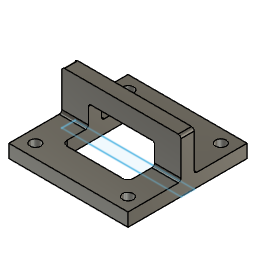
tesion holder v1 (Autodesk Fusion 360 design; units mm, degrees)
Autodesk Fusion 360 part; units mm, degrees
sketch "Sketch1" plane through (0, 0, 0) normal (0, 0, 1) x (1, 0, 0)
  line L0 (0, 0) -> (45, 0)
  line L1 (45, 0) -> (45, 45)
  line L2 (45, 45) -> (0, 45)
  line L3 (0, 45) -> (0, 0)
  line L4 (10, 35) -> (35, 35)
  line L5 (35, 35) -> (35, 10)
  line L6 (35, 10) -> (10, 10)
  line L7 (10, 10) -> (10, 35)
  dimension "d1" = 45
  dimension "d2" = 45
  constraint coincident L0.start L3.end
  constraint horizontal L0
  constraint perpendicular L0 L1
  constraint perpendicular L1 L2
  constraint perpendicular L0 L3
  constraint horizontal L4
  constraint perpendicular L4 L5
  constraint perpendicular L5 L6
  constraint perpendicular L4 L7
  measures "d1" distance of L0.start L0.end
  measures "d2" distance of L0.end L1.end
extrude "Extrude1" add sketch "Sketch1" along normal blind 5
hole "Hole1" at (5.1121, 40.0517, 5) direction (0, 0, -1) diameter 4 depth 10 tip angle 180
hole "Hole2" at (4.9695, 5.025, 5) direction (0, 0, -1) diameter 4 depth 6 tip angle 180
hole "Hole3" at (39.9447, 5.025, 5) direction (0, 0, -1) diameter 4 depth 6 tip angle 180
hole "Hole4" at (40.0084, 40.0762, 5) direction (0, 0, -1) diameter 4 depth 6 tip angle 180
sketch "Sketch2" plane through (0, 0, 0) normal (0, 0, 1) x (1, 0, 0)
  line L0 (45, 25) -> (45, 20)
  line L1 (45, 20) -> (0, 20)
  line L2 (0, 20) -> (0, 25)
  line L3 (0, 25) -> (0, 20)
  line L4 (0, 25) -> (45, 25)
  constraint vertical L0
  constraint perpendicular L0 L1
  constraint perpendicular L1 L2
  constraint perpendicular L0 L4
extrude "Extrude2" add sketch "Sketch2" along normal blind 20
sketch "Sketch4" plane through (0, 25, 0) normal (0, 1, 0) x (-1, 0, 0)
  line L0 (-45, 5) -> (-35, 5)
  line L1 (-35, 5) -> (-35, 0)
  line L2 (-35, 0) -> (-10, 0)
  line L3 (-10, 0) -> (-10, 5)
  line L4 (-10, 5) -> (0, 5)
  line L5 (0, 5) -> (0, 20)
  line L6 (0, 20) -> (-45, 20)
  line L7 (-45, 20) -> (-45, 5)
  line L8 (-10, 0) -> (-35, 0)
  line L9 (-35, 0) -> (-35, 13.0137)
  line L10 (-35, 13.0137) -> (-10, 13.0137)
  line L11 (-10, 13.0137) -> (-10, 0)
  constraint horizontal L8
  constraint vertical L9
  constraint horizontal L10
  constraint vertical L11
  constraint coincident L2.end L3.start
extrude "Extrude3" cut sketch "Sketch4" against normal blind 5 contours L1 L2 L3 L8 L9 L10 L11
fillet "Fillet1" radius 1 1 edges at (35, 22.5, 13.0137)
fillet "Fillet2" radius 1 1 edges at (10, 22.5, 13.0137)
fillet "Fillet3" radius 1 1 edges at (45, 22.5, 20)
fillet "Fillet4" radius 1 1 edges at (0, 22.5, 20)
fillet "Fillet5" radius 1 1 edges at (40, 20, 5)
fillet "Fillet6" radius 1 1 edges at (40, 25, 5)
fillet "Fillet7" radius 1 1 edges at (5, 20, 5)
fillet "Fillet8" radius 1 1 edges at (5, 25, 5)
fillet "Fillet9" radius 2 1 edges at (35, 35, 2.5)
fillet "Fillet10" radius 2 1 edges at (10, 35, 2.5)
fillet "Fillet11" radius 2 1 edges at (10, 10, 2.5)
fillet "Fillet12" radius 2 1 edges at (35, 10, 2.5)
